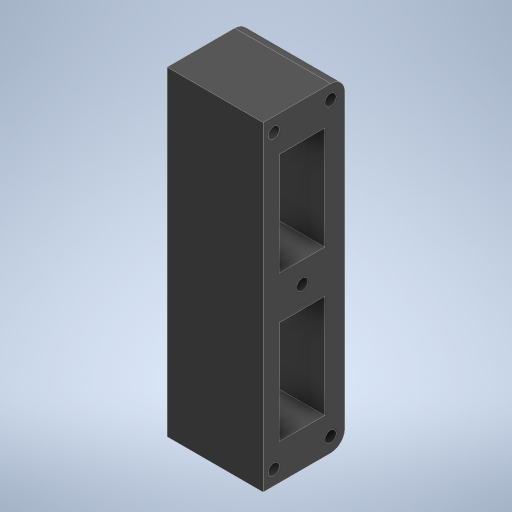
# Autodesk Inventor part: chest_cover_stopper
Saved by Autodesk Inventor 2024.1 (Build 281209000, 209)
## iProperties
Created: 2024-02-15
Part Number: chest_cover_stopper
Material: 一般
Document SubType Name: Modeling
Designer: hibik
Density: 1 g/cm^3
Appearance: 既定
Author: hibik
Autodesk Inventor part; units mm, degrees
ref_plane "YZ Plane" through (0, 0, 0) normal (1, 0, 0) x (0, 1, 0)
ref_plane "XZ Plane" through (0, 0, 0) normal (0, 1, 0) x (-1, 0, 0)
ref_plane "XY Plane" through (0, 0, 0) normal (0, 0, 1) x (1, 0, 0)
sketch "スケッチ1" plane through (0, 0, 0) normal (1, 0, 0) x (0, 1, 0)
  line L0 (45, 0) -> (0, 0)
  line L1 (0, 0) -> (0, -11.5)
  line L2 (0, -11.5) -> (45, -11.5)
  line L3 (45, -11.5) -> (45, 0)
  dimension "d0" = 45
  dimension "d1" = 11.5
  constraints: 8 end point, 2 parallel, 1 coincident, 1 horizontal, 1 perpendicular
  measures "d0" distance of L0.start L0.end
  measures "d1" distance of L2.end L0.start
extrude "押し出し1" add sketch "スケッチ1" along normal blind 13.5
sketch "スケッチ2" plane through (13.5, 0, 0) normal (1, 0, 0) x (0, 0, -1)
  circle A0 centre (1.5, 43) radius 0.8 projected
  circle A1 centre (9.4807, 43) radius 0.8 projected
  circle A2 centre (9.5, 2) radius 0.8 projected
  circle A3 centre (1.5, 2) radius 0.8 projected
  circle A4 centre (5.5, 22.5) radius 0.8 projected
  point P0 (0, 0)
extrude "押し出し2" cut sketch "スケッチ2" against normal through all
fillet "フィレット1" radius 2 2 edges at (6.75, 45, -11.5) (6.75, 0, -11.5)
sketch "スケッチ4" plane through (13.5, 0, 0) normal (1, 0, 0) x (0, 0, -1)
  line L0 (2.3, 40) -> (8.6807, 40)
  line L1 (8.6807, 40) -> (8.6807, 25.5)
  line L2 (8.6807, 25.5) -> (2.3, 25.5)
  line L3 (2.3, 25.5) -> (2.3, 40)
  line L4 (2.3, 19.5) -> (8.6807, 19.5)
  line L5 (8.6807, 19.5) -> (8.6807, 5)
  line L6 (8.6807, 5) -> (2.3, 5)
  line L7 (2.3, 5) -> (2.3, 19.5)
  circle A0 centre (1.5, 43) radius 0.8 projected
  arc A1 (9.5, 0) -> (11.5, 2) centre (9.5, 2) ccw projected
  line L8 (11.5, 2) -> (11.5, 43) projected
  arc A2 (11.5, 43) -> (9.5, 45) centre (9.5, 43) ccw projected
  line L9 (9.5, 45) -> (0, 45) projected
  line L10 (0, 45) -> (0, 0) projected
  line L11 (0, 0) -> (9.5, 0) projected
  circle A3 centre (5.5, 22.5) radius 0.8 projected
  circle A4 centre (9.5, 2) radius 0.8 projected
  circle A5 centre (1.5, 2) radius 0.8 projected
  circle A6 centre (9.4807, 43) radius 0.8 projected
  circle A7 centre (1.5, 43) radius 0.8 projected
  dimension "d9" = 3
  dimension "d10" = 3
  dimension "d11" = 3
  dimension "d12" = 3
  constraints: 16 end point, 4 parallel, 2 horizontal, 2 perpendicular, 2 tangent, 1 collinear, 1 point on line
  measures "d9" distance from line of A3.centre L2
  measures "d10" distance from line of A0.centre L0
  measures "d11" distance from line of L4 A3.centre
  measures "d12" distance from line of A1.centre L6
extrude "押し出し3" cut sketch "スケッチ4" against normal through all contours L0 L1 L2 L3 | L4 L5 L6 L7
